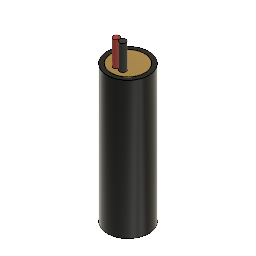
Laser Diode (Autodesk Fusion 360 design; units mm, degrees)
Autodesk Fusion 360 part; units mm, degrees
note: some values were not read from the file. Set by a fixed rule: which sketch regions a step uses; which face or edge a step refers to.
sketch "Sketch1" plane through (0, 0, 0) normal (0, 0, 1) x (1, 0, 0)
  circle A0 centre (0, 0) radius 5
  circle A1 centre (0, 0) radius 3.4
  circle A2 centre (0, 0) radius 1.5
  line L0 (-4, -0.5) -> (4, -0.5)
  line L1 (4, -0.5) -> (4, 0.5)
  line L2 (4, 0.5) -> (-4, 0.5)
  line L3 (-4, 0.5) -> (-4, -0.5)
  line L4 (0, 0.5) -> (0, 0) construction
  line L5 (4, 0) -> (0, 0) construction
  circle A3 centre (0, 0) radius 4
  dimension "d1" = 10
  dimension "d2" = 6.8
  dimension "d3" = 3
  dimension "d4" = 1
  dimension "d5" = 8
  dimension "d20" = 8
  constraint coincident A0.centre A1.centre
  constraint concentric A0 A2
  constraint horizontal L0
  constraint vertical L1
  constraint horizontal L2
  constraint vertical L3
  constraint midpoint L2 L4.start
  constraint perpendicular L2 L4
  constraint midpoint L1 L5.start
  constraint perpendicular L1 L5
  measures "d1" diameter of A0
  measures "d2" diameter of A1
  measures "d3" diameter of A2
  measures "d4" distance of L0.end L1.end
  measures "d5" distance of L1.end L2.end
  measures "d20" diameter of A3
extrude "Extrude1" add sketch "Sketch1" along normal blind 32.8 contours A0 | L1 L2 A3 | L0 L1 A3 | L2 L3 A3 | L0 L3 A3 makes body 1
extrude "Extrude2" add sketch "Sketch1" along normal blind 32.8 separate body contours A1 A2 L0 L2 | A1 L0 L2 A3 | A1 A2 L2 | A1 L2 A3 | A1 L0 A3 | A1 A2 L0 | A1 A2 L0 L2 | A1 L0 L2 A3 | A2 L2 | A2 L0 L2 | A2 L0 makes body 2
sketch "Sketch3" plane through (0, 0, 0) normal (1, 0, 0) x (0, 1, 0)
  line L0 (3.4, 0) -> (-3.4, 0)
  line L1 (2.9, 0) -> (3.4, 0.5)
  line L2 (3.4, 0.5) -> (3.9, 0)
  line L3 (3.9, 0) -> (2.9, 0)
  dimension "d13" = 1
  dimension "d14" = 45
  constraint parallel L0 L3
  constraint perpendicular L1 L2
  constraint midpoint L0.start L3
  measures "d13" distance of L1.start L2.end
  measures "d14" angle of L1 L3
revolve "Revolve1" cut sketch "Sketch3" angle 360 about axis through (0, 0, 0) along (0, 0, -1) bodies 2
extrude "Extrude3" cut sketch "Sketch1" along normal blind 1.2 contours A2 L2 | A2 L0 L2 | A2 L0 bodies 2
extrude "Extrude4" cut sketch "Sketch1" along normal blind 0.5 contours A1 A2 L0 L2 | A1 A2 L0 L2 | L1 L2 A3 | A2 L0 L2 | L0 L1 A3 | L2 L3 A3 | L0 L3 A3 bodies 2
extrude "Extrude5" add sketch "Sketch1" along normal blind 1 separate body contours A2 L2 | A2 L0 L2 | A2 L0 makes body 3
move_face "OffsetFaces1" offset -0.1 1 faces at (1.0205, -1.0993, 0.6667) on bodies 3
fillet "Fillet1" radius 0.6 1 edges at (-1.3053, -0.5063, 0) on bodies 3
chamfer "Chamfer1" distance 0.2 angle 45 2 edges at (0, -1.5, 0) (0, 1.5, 0) on bodies 2
sketch "Sketch4" plane through (0, 0, 32.8) normal (0, 0, 1) x (-1, 0, 0)
  circle A0 centre (0.75, 2) radius 0.75
  line L0 (0, 0) -> (0, -3) construction
  circle A1 centre (-0.75, 2) radius 0.75
  dimension "d26" = 1.5
  dimension "d27" = 0.75
  dimension "d28" = 2
  constraint coincident L0.start origin
  constraint vertical L0
  constraint symmetric A0 L0 A1
  measures "d26" diameter of A0
  measures "d27" horizontal distance of L0.start A0.centre
  measures "d28" vertical distance of L0.start A0.centre
extrude "Extrude6" add sketch "Sketch4" along normal blind 6 separate body contours A0 makes body 4
extrude "Extrude7" add sketch "Sketch4" along normal blind 6 separate body contours A1 makes body 5
equation "d9 = length"
equation "d11 = length"
equation "length = 32.8 mm"
